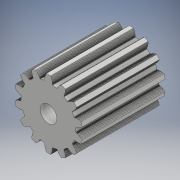
# Autodesk Inventor part: engranaje_pequeño_1
Saved by Autodesk Inventor 2017 (Build 210142000, 142)
## iProperties
Created: 2016-10-04
Part Number: engranaje_pequeño_1
Material: Generic
Document SubType Name: Modeling
Designer: ANDRES
Density: 1 g/cm^3
Appearance: Default
Author: ANDRES
Autodesk Inventor part; units mm, degrees
(part 1 of 2)
ref_plane "YZ Plane" through (0, 0, 0) normal (1, 0, 0) x (0, 1, 0)
ref_plane "XZ Plane" through (0, 0, 0) normal (0, 1, 0) x (-1, 0, 0)
ref_plane "XY Plane" through (0, 0, 0) normal (0, 0, 1) x (1, 0, 0)
sketch "Sketch1" plane through (0, 0, 0) normal (0, 1, 0) x (-1, 0, 0)
  line L0 (0.0808, 0.4341) -> (0.0797, 0.4378)
  line L1 (0.0797, 0.4378) -> (0.0785, 0.4393)
  line L2 (0.0785, 0.4393) -> (0.0772, 0.4404)
  line L3 (0.0772, 0.4404) -> (0.076, 0.4413)
  line L4 (0.076, 0.4413) -> (0.0747, 0.442)
  line L5 (0.0747, 0.442) -> (0.0734, 0.4426)
  line L6 (0.0734, 0.4426) -> (0.0708, 0.4437)
  line L7 (0.0708, 0.4437) -> (0.0682, 0.4445)
  line L8 (0.0682, 0.4445) -> (0.0656, 0.4451)
  line L9 (0.0656, 0.4451) -> (0.0604, 0.4462)
  line L10 (0.0604, 0.4462) -> (0.0552, 0.4478)
  line L11 (0.0552, 0.4478) -> (0.05, 0.4497)
  line L12 (0.05, 0.4497) -> (0.0449, 0.452)
  line L13 (0.0449, 0.452) -> (0.0398, 0.4545)
  line L14 (0.0398, 0.4545) -> (0.0348, 0.4573)
  line L15 (0.0348, 0.4573) -> (0.0298, 0.4603)
  line L16 (0.0298, 0.4603) -> (0.0248, 0.4636)
  line L17 (0.0248, 0.4636) -> (0.0199, 0.467)
  line L18 (0.0199, 0.467) -> (0.015, 0.4707)
  line L19 (0.015, 0.4707) -> (0.0102, 0.4745)
  line L20 (0.0102, 0.4745) -> (0.0055, 0.4786)
  line L21 (0.0055, 0.4786) -> (0.0167, 0.5276)
  line L22 (0.0167, 0.5276) -> (0.0227, 0.5292)
  line L23 (0.0227, 0.5292) -> (0.0287, 0.5306)
  line L24 (0.0287, 0.5306) -> (0.0347, 0.5318)
  line L25 (0.0347, 0.5318) -> (0.0406, 0.5328)
  line L26 (0.0406, 0.5328) -> (0.0465, 0.5335)
  line L27 (0.0465, 0.5335) -> (0.0523, 0.5341)
  line L28 (0.0523, 0.5341) -> (0.058, 0.5344)
  line L29 (0.058, 0.5344) -> (0.0637, 0.5345)
  line L30 (0.0637, 0.5345) -> (0.0693, 0.5343)
  line L31 (0.0693, 0.5343) -> (0.0748, 0.5338)
  line L32 (0.0748, 0.5338) -> (0.0802, 0.5329)
  line L33 (0.0802, 0.5329) -> (0.0854, 0.5316)
  line L34 (0.0854, 0.5316) -> (0.088, 0.5311)
  line L35 (0.088, 0.5311) -> (0.0907, 0.5307)
  line L36 (0.0907, 0.5307) -> (0.0935, 0.5305)
  line L37 (0.0935, 0.5305) -> (0.0949, 0.5305)
  line L38 (0.0949, 0.5305) -> (0.0964, 0.5307)
  line L39 (0.0964, 0.5307) -> (0.0979, 0.5309)
  line L40 (0.0979, 0.5309) -> (0.0995, 0.5313)
  line L41 (0.0995, 0.5313) -> (0.1012, 0.5322)
  line L42 (0.1012, 0.5322) -> (0.1038, 0.535)
  line L43 (0.1038, 0.535) -> (0.1233, 0.5755)
  line L44 (0.1233, 0.5755) -> (0.1239, 0.5792)
  line L45 (0.1239, 0.5792) -> (0.1235, 0.5811)
  line L46 (0.1235, 0.5811) -> (0.1228, 0.5826)
  line L47 (0.1228, 0.5826) -> (0.1221, 0.584)
  line L48 (0.1221, 0.584) -> (0.1212, 0.5852)
  line L49 (0.1212, 0.5852) -> (0.1204, 0.5863)
  line L50 (0.1204, 0.5863) -> (0.1185, 0.5884)
  line L51 (0.1185, 0.5884) -> (0.1165, 0.5903)
  line L52 (0.1165, 0.5903) -> (0.1144, 0.592)
  line L53 (0.1144, 0.592) -> (0.1102, 0.5952)
  line L54 (0.1102, 0.5952) -> (0.1061, 0.5989)
  line L55 (0.1061, 0.5989) -> (0.1023, 0.6029)
  line L56 (0.1023, 0.6029) -> (0.0987, 0.6071)
  line L57 (0.0987, 0.6071) -> (0.0952, 0.6116)
  line L58 (0.0952, 0.6116) -> (0.0919, 0.6163)
  line L59 (0.0919, 0.6163) -> (0.0887, 0.6212)
  line L60 (0.0887, 0.6212) -> (0.0856, 0.6263)
  line L61 (0.0856, 0.6263) -> (0.0827, 0.6315)
  line L62 (0.0827, 0.6315) -> (0.0799, 0.6369)
  line L63 (0.0799, 0.6369) -> (0.0773, 0.6425)
  line L64 (0.0773, 0.6425) -> (0.0747, 0.6482)
  line L65 (0.0747, 0.6482) -> (0.1061, 0.6875)
  line L66 (0.1061, 0.6875) -> (0.1122, 0.6863)
  line L67 (0.1122, 0.6863) -> (0.1182, 0.685)
  line L68 (0.1182, 0.685) -> (0.1241, 0.6835)
  line L69 (0.1241, 0.6835) -> (0.1299, 0.6818)
  line L70 (0.1299, 0.6818) -> (0.1355, 0.6799)
  line L71 (0.1355, 0.6799) -> (0.141, 0.6779)
  line L72 (0.141, 0.6779) -> (0.1463, 0.6757)
  line L73 (0.1463, 0.6757) -> (0.1515, 0.6733)
  line L74 (0.1515, 0.6733) -> (0.1564, 0.6707)
  line L75 (0.1564, 0.6707) -> (0.1612, 0.6679)
  line L76 (0.1612, 0.6679) -> (0.1656, 0.6648)
  line L77 (0.1656, 0.6648) -> (0.1697, 0.6613)
  line L78 (0.1697, 0.6613) -> (0.1719, 0.6597)
  line L79 (0.1719, 0.6597) -> (0.1741, 0.6582)
  line L80 (0.1741, 0.6582) -> (0.1766, 0.6568)
  line L81 (0.1766, 0.6568) -> (0.1779, 0.6562)
  line L82 (0.1779, 0.6562) -> (0.1792, 0.6557)
  line L83 (0.1792, 0.6557) -> (0.1807, 0.6552)
  line L84 (0.1807, 0.6552) -> (0.1823, 0.6549)
  line L85 (0.1823, 0.6549) -> (0.1843, 0.6549)
  line L86 (0.1843, 0.6549) -> (0.1878, 0.6564)
  line L87 (0.1878, 0.6564) -> (0.2229, 0.6844)
  line L88 (0.2229, 0.6844) -> (0.2251, 0.6875)
  line L89 (0.2251, 0.6875) -> (0.2255, 0.6894)
  line L90 (0.2255, 0.6894) -> (0.2256, 0.691)
  line L91 (0.2256, 0.691) -> (0.2255, 0.6926)
  line L92 (0.2255, 0.6926) -> (0.2253, 0.694)
  line L93 (0.2253, 0.694) -> (0.225, 0.6954)
  line L94 (0.225, 0.6954) -> (0.2242, 0.6981)
  line L95 (0.2242, 0.6981) -> (0.2232, 0.7006)
  line L96 (0.2232, 0.7006) -> (0.2221, 0.7031)
  line L97 (0.2221, 0.7031) -> (0.2197, 0.7079)
  line L98 (0.2197, 0.7079) -> (0.2176, 0.7129)
  line L99 (0.2176, 0.7129) -> (0.2159, 0.7182)
  line L100 (0.2159, 0.7182) -> (0.2145, 0.7236)
  line L101 (0.2145, 0.7236) -> (0.2133, 0.7291)
  line L102 (0.2133, 0.7291) -> (0.2123, 0.7348)
  line L103 (0.2123, 0.7348) -> (0.2116, 0.7406)
  line L104 (0.2116, 0.7406) -> (0.211, 0.7465)
  line L105 (0.211, 0.7465) -> (0.2107, 0.7525)
  line L106 (0.2107, 0.7525) -> (0.2105, 0.7586)
  line L107 (0.2105, 0.7586) -> (0.2105, 0.7647)
  line L108 (0.2105, 0.7647) -> (0.2107, 0.771)
  line L109 (0.2107, 0.771) -> (0.256, 0.7928)
  line L110 (0.256, 0.7928) -> (0.261, 0.7891)
  line L111 (0.261, 0.7891) -> (0.2659, 0.7852)
  line L112 (0.2659, 0.7852) -> (0.2705, 0.7813)
  line L113 (0.2705, 0.7813) -> (0.275, 0.7773)
  line L114 (0.275, 0.7773) -> (0.2793, 0.7732)
  line L115 (0.2793, 0.7732) -> (0.2833, 0.769)
  line L116 (0.2833, 0.769) -> (0.2872, 0.7647)
  line L117 (0.2872, 0.7647) -> (0.2908, 0.7603)
  line L118 (0.2908, 0.7603) -> (0.2941, 0.7558)
  line L119 (0.2941, 0.7558) -> (0.2971, 0.7512)
  line L120 (0.2971, 0.7512) -> (0.2998, 0.7465)
  line L121 (0.2998, 0.7465) -> (0.302, 0.7416)
  line L122 (0.302, 0.7416) -> (0.3032, 0.7392)
  line L123 (0.3032, 0.7392) -> (0.3046, 0.7368)
  line L124 (0.3046, 0.7368) -> (0.3062, 0.7345)
  line L125 (0.3062, 0.7345) -> (0.3071, 0.7334)
  line L126 (0.3071, 0.7334) -> (0.3081, 0.7323)
  line L127 (0.3081, 0.7323) -> (0.3093, 0.7313)
  line L128 (0.3093, 0.7313) -> (0.3106, 0.7304)
  line L129 (0.3106, 0.7304) -> (0.3123, 0.7295)
  line L130 (0.3123, 0.7295) -> (0.3161, 0.7293)
  line L131 (0.3161, 0.7293) -> (0.3599, 0.7393)
  line L132 (0.3599, 0.7393) -> (0.3633, 0.7411)
  line L133 (0.3633, 0.7411) -> (0.3644, 0.7426)
  line L134 (0.3644, 0.7426) -> (0.3652, 0.7441)
  line L135 (0.3652, 0.7441) -> (0.3658, 0.7455)
  line L136 (0.3658, 0.7455) -> (0.3663, 0.7469)
  line L137 (0.3663, 0.7469) -> (0.3666, 0.7483)
  line L138 (0.3666, 0.7483) -> (0.367, 0.7511)
  line L139 (0.367, 0.7511) -> (0.3673, 0.7538)
  line L140 (0.3673, 0.7538) -> (0.3673, 0.7565)
  line L141 (0.3673, 0.7565) -> (0.3672, 0.7618)
  line L142 (0.3672, 0.7618) -> (0.3676, 0.7673)
  line L143 (0.3676, 0.7673) -> (0.3683, 0.7727)
  line L144 (0.3683, 0.7727) -> (0.3694, 0.7782)
  line L145 (0.3694, 0.7782) -> (0.3707, 0.7837)
  line L146 (0.3707, 0.7837) -> (0.3723, 0.7893)
  line L147 (0.3723, 0.7893) -> (0.3741, 0.7948)
  line L148 (0.3741, 0.7948) -> (0.3762, 0.8004)
  line L149 (0.3762, 0.8004) -> (0.3784, 0.8059)
  line L150 (0.3784, 0.8059) -> (0.3809, 0.8115)
  line L151 (0.3809, 0.8115) -> (0.3836, 0.817)
  line L152 (0.3836, 0.817) -> (0.3865, 0.8226)
  line L153 (0.3865, 0.8226) -> (0.4368, 0.8226)
  line L154 (0.4368, 0.8226) -> (0.4397, 0.817)
  line L155 (0.4397, 0.817) -> (0.4424, 0.8115)
  line L156 (0.4424, 0.8115) -> (0.4449, 0.8059)
  line L157 (0.4449, 0.8059) -> (0.4472, 0.8004)
  line L158 (0.4472, 0.8004) -> (0.4492, 0.7948)
  line L159 (0.4492, 0.7948) -> (0.4511, 0.7893)
  line L160 (0.4511, 0.7893) -> (0.4526, 0.7837)
  line L161 (0.4526, 0.7837) -> (0.454, 0.7782)
  line L162 (0.454, 0.7782) -> (0.455, 0.7727)
  line L163 (0.455, 0.7727) -> (0.4558, 0.7673)
  line L164 (0.4558, 0.7673) -> (0.4561, 0.7618)
  line L165 (0.4561, 0.7618) -> (0.456, 0.7565)
  line L166 (0.456, 0.7565) -> (0.4561, 0.7538)
  line L167 (0.4561, 0.7538) -> (0.4563, 0.7511)
  line L168 (0.4563, 0.7511) -> (0.4567, 0.7483)
  line L169 (0.4567, 0.7483) -> (0.4571, 0.7469)
  line L170 (0.4571, 0.7469) -> (0.4575, 0.7455)
  line L171 (0.4575, 0.7455) -> (0.4581, 0.7441)
  line L172 (0.4581, 0.7441) -> (0.4589, 0.7426)
  line L173 (0.4589, 0.7426) -> (0.4601, 0.7411)
  line L174 (0.4601, 0.7411) -> (0.4634, 0.7393)
  line L175 (0.4634, 0.7393) -> (0.5072, 0.7293)
  line L176 (0.5072, 0.7293) -> (0.511, 0.7295)
  line L177 (0.511, 0.7295) -> (0.5127, 0.7304)
  line L178 (0.5127, 0.7304) -> (0.5141, 0.7313)
  line L179 (0.5141, 0.7313) -> (0.5152, 0.7323)
  line L180 (0.5152, 0.7323) -> (0.5162, 0.7334)
  line L181 (0.5162, 0.7334) -> (0.5171, 0.7345)
  line L182 (0.5171, 0.7345) -> (0.5187, 0.7368)
  line L183 (0.5187, 0.7368) -> (0.5201, 0.7392)
  line L184 (0.5201, 0.7392) -> (0.5213, 0.7416)
  line L185 (0.5213, 0.7416) -> (0.5235, 0.7465)
  line L186 (0.5235, 0.7465) -> (0.5262, 0.7512)
  line L187 (0.5262, 0.7512) -> (0.5292, 0.7558)
  line L188 (0.5292, 0.7558) -> (0.5326, 0.7603)
  line L189 (0.5326, 0.7603) -> (0.5362, 0.7647)
  line L190 (0.5362, 0.7647) -> (0.54, 0.769)
  line L191 (0.54, 0.769) -> (0.5441, 0.7732)
  line L192 (0.5441, 0.7732) -> (0.5483, 0.7773)
  line L193 (0.5483, 0.7773) -> (0.5528, 0.7813)
  line L194 (0.5528, 0.7813) -> (0.5575, 0.7852)
  line L195 (0.5575, 0.7852) -> (0.5623, 0.7891)
  line L196 (0.5623, 0.7891) -> (0.5673, 0.7928)
  line L197 (0.5673, 0.7928) -> (0.6126, 0.771)
  line L198 (0.6126, 0.771) -> (0.6128, 0.7647)
  line L199 (0.6128, 0.7647) -> (0.6128, 0.7586)
  line L200 (0.6128, 0.7586) -> (0.6127, 0.7525)
  line L201 (0.6127, 0.7525) -> (0.6123, 0.7465)
  line L202 (0.6123, 0.7465) -> (0.6118, 0.7406)
  line L203 (0.6118, 0.7406) -> (0.611, 0.7348)
  line L204 (0.611, 0.7348) -> (0.61, 0.7291)
  line L205 (0.61, 0.7291) -> (0.6088, 0.7236)
  line L206 (0.6088, 0.7236) -> (0.6074, 0.7182)
  line L207 (0.6074, 0.7182) -> (0.6057, 0.7129)
  line L208 (0.6057, 0.7129) -> (0.6037, 0.7079)
  line L209 (0.6037, 0.7079) -> (0.6012, 0.7031)
  line L210 (0.6012, 0.7031) -> (0.6001, 0.7006)
  line L211 (0.6001, 0.7006) -> (0.5991, 0.6981)
  line L212 (0.5991, 0.6981) -> (0.5983, 0.6954)
  line L213 (0.5983, 0.6954) -> (0.598, 0.694)
  line L214 (0.598, 0.694) -> (0.5978, 0.6926)
  line L215 (0.5978, 0.6926) -> (0.5977, 0.691)
  line L216 (0.5977, 0.691) -> (0.5978, 0.6894)
  line L217 (0.5978, 0.6894) -> (0.5982, 0.6875)
  line L218 (0.5982, 0.6875) -> (0.6004, 0.6844)
  line L219 (0.6004, 0.6844) -> (0.6355, 0.6564)
  line L220 (0.6355, 0.6564) -> (0.6391, 0.6549)
  line L221 (0.6391, 0.6549) -> (0.641, 0.6549)
  line L222 (0.641, 0.6549) -> (0.6426, 0.6552)
  line L223 (0.6426, 0.6552) -> (0.6441, 0.6557)
  line L224 (0.6441, 0.6557) -> (0.6455, 0.6562)
  line L225 (0.6455, 0.6562) -> (0.6468, 0.6568)
  line L226 (0.6468, 0.6568) -> (0.6492, 0.6582)
  line L227 (0.6492, 0.6582) -> (0.6515, 0.6597)
  line L228 (0.6515, 0.6597) -> (0.6536, 0.6613)
  line L229 (0.6536, 0.6613) -> (0.6577, 0.6648)
  line L230 (0.6577, 0.6648) -> (0.6622, 0.6679)
  line L231 (0.6622, 0.6679) -> (0.6669, 0.6707)
  line L232 (0.6669, 0.6707) -> (0.6719, 0.6733)
  line L233 (0.6719, 0.6733) -> (0.677, 0.6757)
  line L234 (0.677, 0.6757) -> (0.6823, 0.6779)
  line L235 (0.6823, 0.6779) -> (0.6878, 0.6799)
  line L236 (0.6878, 0.6799) -> (0.6934, 0.6818)
  line L237 (0.6934, 0.6818) -> (0.6992, 0.6835)
  line L238 (0.6992, 0.6835) -> (0.7051, 0.685)
  line L239 (0.7051, 0.685) -> (0.7111, 0.6863)
  line L240 (0.7111, 0.6863) -> (0.7172, 0.6875)
  line L241 (0.7172, 0.6875) -> (0.7486, 0.6482)
  line L242 (0.7486, 0.6482) -> (0.7461, 0.6425)
  line L243 (0.7461, 0.6425) -> (0.7434, 0.6369)
  line L244 (0.7434, 0.6369) -> (0.7406, 0.6315)
  line L245 (0.7406, 0.6315) -> (0.7377, 0.6263)
  line L246 (0.7377, 0.6263) -> (0.7347, 0.6212)
  line L247 (0.7347, 0.6212) -> (0.7315, 0.6163)
  line L248 (0.7315, 0.6163) -> (0.7281, 0.6116)
  line L249 (0.7281, 0.6116) -> (0.7246, 0.6071)
  line L250 (0.7246, 0.6071) -> (0.721, 0.6029)
  line L251 (0.721, 0.6029) -> (0.7172, 0.5989)
  line L252 (0.7172, 0.5989) -> (0.7132, 0.5952)
  line L253 (0.7132, 0.5952) -> (0.7089, 0.592)
  line L254 (0.7089, 0.592) -> (0.7068, 0.5903)
  line L255 (0.7068, 0.5903) -> (0.7048, 0.5884)
  line L256 (0.7048, 0.5884) -> (0.703, 0.5863)
  line L257 (0.703, 0.5863) -> (0.7021, 0.5852)
  line L258 (0.7021, 0.5852) -> (0.7013, 0.584)
  line L259 (0.7013, 0.584) -> (0.7005, 0.5826)
  line L260 (0.7005, 0.5826) -> (0.6999, 0.5811)
  line L261 (0.6999, 0.5811) -> (0.6994, 0.5792)
  line L262 (0.6994, 0.5792) -> (0.7, 0.5755)
  line L263 (0.7, 0.5755) -> (0.7195, 0.535)
  line L264 (0.7195, 0.535) -> (0.7221, 0.5322)
  line L265 (0.7221, 0.5322) -> (0.7238, 0.5313)
  line L266 (0.7238, 0.5313) -> (0.7254, 0.5309)
  line L267 (0.7254, 0.5309) -> (0.7269, 0.5307)
  line L268 (0.7269, 0.5307) -> (0.7284, 0.5305)
  line L269 (0.7284, 0.5305) -> (0.7299, 0.5305)
  line L270 (0.7299, 0.5305) -> (0.7326, 0.5307)
  line L271 (0.7326, 0.5307) -> (0.7353, 0.5311)
  line L272 (0.7353, 0.5311) -> (0.738, 0.5316)
  line L273 (0.738, 0.5316) -> (0.7432, 0.5329)
  line L274 (0.7432, 0.5329) -> (0.7485, 0.5338)
  line L275 (0.7485, 0.5338) -> (0.754, 0.5343)
  line L276 (0.754, 0.5343) -> (0.7596, 0.5345)
  line L277 (0.7596, 0.5345) -> (0.7653, 0.5344)
  line L278 (0.7653, 0.5344) -> (0.771, 0.5341)
  line L279 (0.771, 0.5341) -> (0.7769, 0.5335)
  line L280 (0.7769, 0.5335) -> (0.7827, 0.5328)
  line L281 (0.7827, 0.5328) -> (0.7887, 0.5318)
  line L282 (0.7887, 0.5318) -> (0.7946, 0.5306)
  line L283 (0.7946, 0.5306) -> (0.8006, 0.5292)
  line L284 (0.8006, 0.5292) -> (0.8067, 0.5276)
  line L285 (0.8067, 0.5276) -> (0.8178, 0.4786)
  line L286 (0.8178, 0.4786) -> (0.8131, 0.4745)
  line L287 (0.8131, 0.4745) -> (0.8083, 0.4707)
  line L288 (0.8083, 0.4707) -> (0.8034, 0.467)
  line L289 (0.8034, 0.467) -> (0.7985, 0.4636)
  line L290 (0.7985, 0.4636) -> (0.7936, 0.4603)
  line L291 (0.7936, 0.4603) -> (0.7886, 0.4573)
  line L292 (0.7886, 0.4573) -> (0.7835, 0.4545)
  line L293 (0.7835, 0.4545) -> (0.7784, 0.452)
  line L294 (0.7784, 0.452) -> (0.7733, 0.4497)
  line L295 (0.7733, 0.4497) -> (0.7682, 0.4478)
  line L296 (0.7682, 0.4478) -> (0.763, 0.4462)
  line L297 (0.763, 0.4462) -> (0.7577, 0.4451)
  line L298 (0.7577, 0.4451) -> (0.7551, 0.4445)
  line L299 (0.7551, 0.4445) -> (0.7525, 0.4437)
  line L300 (0.7525, 0.4437) -> (0.7499, 0.4426)
  line L301 (0.7499, 0.4426) -> (0.7486, 0.442)
  line L302 (0.7486, 0.442) -> (0.7473, 0.4413)
  line L303 (0.7473, 0.4413) -> (0.7461, 0.4404)
  line L304 (0.7461, 0.4404) -> (0.7449, 0.4393)
  line L305 (0.7449, 0.4393) -> (0.7436, 0.4378)
  line L306 (0.7436, 0.4378) -> (0.7426, 0.4341)
  line L307 (0.7426, 0.4341) -> (0.7426, 0.3892)
  line L308 (0.7426, 0.3892) -> (0.7436, 0.3855)
  line L309 (0.7436, 0.3855) -> (0.7449, 0.3841)
  line L310 (0.7449, 0.3841) -> (0.7461, 0.383)
  line L311 (0.7461, 0.383) -> (0.7473, 0.3821)
  line L312 (0.7473, 0.3821) -> (0.7486, 0.3813)
  line L313 (0.7486, 0.3813) -> (0.7499, 0.3807)
  line L314 (0.7499, 0.3807) -> (0.7525, 0.3796)
  line L315 (0.7525, 0.3796) -> (0.7551, 0.3788)
  line L316 (0.7551, 0.3788) -> (0.7577, 0.3782)
  line L317 (0.7577, 0.3782) -> (0.763, 0.3771)
  line L318 (0.763, 0.3771) -> (0.7682, 0.3755)
  line L319 (0.7682, 0.3755) -> (0.7733, 0.3736)
  line L320 (0.7733, 0.3736) -> (0.7784, 0.3714)
  line L321 (0.7784, 0.3714) -> (0.7835, 0.3688)
  line L322 (0.7835, 0.3688) -> (0.7886, 0.366)
  line L323 (0.7886, 0.366) -> (0.7936, 0.363)
  line L324 (0.7936, 0.363) -> (0.7985, 0.3598)
  line L325 (0.7985, 0.3598) -> (0.8034, 0.3563)
  line L326 (0.8034, 0.3563) -> (0.8083, 0.3527)
  line L327 (0.8083, 0.3527) -> (0.8131, 0.3488)
  line L328 (0.8131, 0.3488) -> (0.8178, 0.3447)
  line L329 (0.8178, 0.3447) -> (0.8067, 0.2957)
  line L330 (0.8067, 0.2957) -> (0.8006, 0.2941)
  line L331 (0.8006, 0.2941) -> (0.7946, 0.2927)
  line L332 (0.7946, 0.2927) -> (0.7887, 0.2915)
  line L333 (0.7887, 0.2915) -> (0.7827, 0.2906)
  line L334 (0.7827, 0.2906) -> (0.7769, 0.2898)
  line L335 (0.7769, 0.2898) -> (0.771, 0.2892)
  line L336 (0.771, 0.2892) -> (0.7653, 0.2889)
  line L337 (0.7653, 0.2889) -> (0.7596, 0.2888)
  line L338 (0.7596, 0.2888) -> (0.754, 0.289)
  line L339 (0.754, 0.289) -> (0.7485, 0.2895)
  line L340 (0.7485, 0.2895) -> (0.7432, 0.2904)
  line L341 (0.7432, 0.2904) -> (0.738, 0.2917)
  line L342 (0.738, 0.2917) -> (0.7353, 0.2923)
  line L343 (0.7353, 0.2923) -> (0.7326, 0.2927)
  line L344 (0.7326, 0.2927) -> (0.7299, 0.2928)
  line L345 (0.7299, 0.2928) -> (0.7284, 0.2928)
  line L346 (0.7284, 0.2928) -> (0.7269, 0.2927)
  line L347 (0.7269, 0.2927) -> (0.7254, 0.2924)
  line L348 (0.7254, 0.2924) -> (0.7238, 0.292)
  line L349 (0.7238, 0.292) -> (0.7221, 0.2912)
  line L350 (0.7221, 0.2912) -> (0.7195, 0.2883)
  line L351 (0.7195, 0.2883) -> (0.7, 0.2479)
  line L352 (0.7, 0.2479) -> (0.6994, 0.2441)
  line L353 (0.6994, 0.2441) -> (0.6999, 0.2422)
  line L354 (0.6999, 0.2422) -> (0.7005, 0.2407)
  line L355 (0.7005, 0.2407) -> (0.7013, 0.2394)
  line L356 (0.7013, 0.2394) -> (0.7021, 0.2381)
  line L357 (0.7021, 0.2381) -> (0.703, 0.237)
  line L358 (0.703, 0.237) -> (0.7048, 0.2349)
  line L359 (0.7048, 0.2349) -> (0.7068, 0.2331)
  line L360 (0.7068, 0.2331) -> (0.7089, 0.2314)
  line L361 (0.7089, 0.2314) -> (0.7132, 0.2281)
  line L362 (0.7132, 0.2281) -> (0.7172, 0.2244)
  line L363 (0.7172, 0.2244) -> (0.721, 0.2205)
  line L364 (0.721, 0.2205) -> (0.7246, 0.2162)
  line L365 (0.7246, 0.2162) -> (0.7281, 0.2117)
  line L366 (0.7281, 0.2117) -> (0.7315, 0.207)
  line L367 (0.7315, 0.207) -> (0.7347, 0.2021)
  line L368 (0.7347, 0.2021) -> (0.7377, 0.1971)
  line L369 (0.7377, 0.1971) -> (0.7406, 0.1918)
  line L370 (0.7406, 0.1918) -> (0.7434, 0.1864)
  line L371 (0.7434, 0.1864) -> (0.7461, 0.1809)
  line L372 (0.7461, 0.1809) -> (0.7486, 0.1751)
  line L373 (0.7486, 0.1751) -> (0.7172, 0.1358)
  line L374 (0.7172, 0.1358) -> (0.7111, 0.137)
  line L375 (0.7111, 0.137) -> (0.7051, 0.1384)
  line L376 (0.7051, 0.1384) -> (0.6992, 0.1399)
  line L377 (0.6992, 0.1399) -> (0.6934, 0.1416)
  line L378 (0.6934, 0.1416) -> (0.6878, 0.1434)
  line L379 (0.6878, 0.1434) -> (0.6823, 0.1454)
  line L380 (0.6823, 0.1454) -> (0.677, 0.1476)
  line L381 (0.677, 0.1476) -> (0.6719, 0.15)
  line L382 (0.6719, 0.15) -> (0.6669, 0.1526)
  line L383 (0.6669, 0.1526) -> (0.6622, 0.1555)
  line L384 (0.6622, 0.1555) -> (0.6577, 0.1586)
  line L385 (0.6577, 0.1586) -> (0.6536, 0.162)
  line L386 (0.6536, 0.162) -> (0.6515, 0.1637)
  line L387 (0.6515, 0.1637) -> (0.6492, 0.1652)
  line L388 (0.6492, 0.1652) -> (0.6468, 0.1665)
  line L389 (0.6468, 0.1665) -> (0.6455, 0.1671)
  line L390 (0.6455, 0.1671) -> (0.6441, 0.1677)
  line L391 (0.6441, 0.1677) -> (0.6426, 0.1681)
  line L392 (0.6426, 0.1681) -> (0.641, 0.1684)
  line L393 (0.641, 0.1684) -> (0.6391, 0.1684)
  line L394 (0.6391, 0.1684) -> (0.6355, 0.167)
  line L395 (0.6355, 0.167) -> (0.6004, 0.1389)
  line L396 (0.6004, 0.1389) -> (0.5982, 0.1358)
  line L397 (0.5982, 0.1358) -> (0.5978, 0.134)
  line L398 (0.5978, 0.134) -> (0.5977, 0.1323)
  line L399 (0.5977, 0.1323) -> (0.5978, 0.1308)
  line L400 (0.5978, 0.1308) -> (0.598, 0.1293)
  line L401 (0.598, 0.1293) -> (0.5983, 0.1279)
  line L402 (0.5983, 0.1279) -> (0.5991, 0.1252)
  line L403 (0.5991, 0.1252) -> (0.6001, 0.1227)
  line L404 (0.6001, 0.1227) -> (0.6012, 0.1203)
  line L405 (0.6012, 0.1203) -> (0.6037, 0.1155)
  line L406 (0.6037, 0.1155) -> (0.6057, 0.1104)
  line L407 (0.6057, 0.1104) -> (0.6074, 0.1052)
  line L408 (0.6074, 0.1052) -> (0.6088, 0.0998)
  line L409 (0.6088, 0.0998) -> (0.61, 0.0942)
  line L410 (0.61, 0.0942) -> (0.611, 0.0885)
  line L411 (0.611, 0.0885) -> (0.6118, 0.0828)
  line L412 (0.6118, 0.0828) -> (0.6123, 0.0769)
  line L413 (0.6123, 0.0769) -> (0.6127, 0.0709)
  line L414 (0.6127, 0.0709) -> (0.6128, 0.0648)
  line L415 (0.6128, 0.0648) -> (0.6128, 0.0586)
  line L416 (0.6128, 0.0586) -> (0.6126, 0.0524)
  line L417 (0.6126, 0.0524) -> (0.5673, 0.0306)
  line L418 (0.5673, 0.0306) -> (0.5623, 0.0343)
  line L419 (0.5623, 0.0343) -> (0.5575, 0.0381)
  line L420 (0.5575, 0.0381) -> (0.5528, 0.042)
  line L421 (0.5528, 0.042) -> (0.5483, 0.046)
  line L422 (0.5483, 0.046) -> (0.5441, 0.0502)
  line L423 (0.5441, 0.0502) -> (0.54, 0.0544)
  line L424 (0.54, 0.0544) -> (0.5362, 0.0587)
  line L425 (0.5362, 0.0587) -> (0.5326, 0.063)
  line L426 (0.5326, 0.063) -> (0.5292, 0.0675)
  line L427 (0.5292, 0.0675) -> (0.5262, 0.0721)
  line L428 (0.5262, 0.0721) -> (0.5235, 0.0769)
  line L429 (0.5235, 0.0769) -> (0.5213, 0.0818)
  line L430 (0.5213, 0.0818) -> (0.5201, 0.0842)
  line L431 (0.5201, 0.0842) -> (0.5187, 0.0865)
  line L432 (0.5187, 0.0865) -> (0.5171, 0.0888)
  line L433 (0.5171, 0.0888) -> (0.5162, 0.0899)
  line L434 (0.5162, 0.0899) -> (0.5152, 0.091)
  line L435 (0.5152, 0.091) -> (0.5141, 0.092)
  line L436 (0.5141, 0.092) -> (0.5127, 0.093)
  line L437 (0.5127, 0.093) -> (0.511, 0.0938)
  line L438 (0.511, 0.0938) -> (0.5072, 0.0941)
  line L439 (0.5072, 0.0941) -> (0.4634, 0.0841)
  line L440 (0.4634, 0.0841) -> (0.4601, 0.0822)
  line L441 (0.4601, 0.0822) -> (0.4589, 0.0807)
  line L442 (0.4589, 0.0807) -> (0.4581, 0.0792)
  line L443 (0.4581, 0.0792) -> (0.4575, 0.0778)
  line L444 (0.4575, 0.0778) -> (0.4571, 0.0764)
  line L445 (0.4571, 0.0764) -> (0.4567, 0.075)
  line L446 (0.4567, 0.075) -> (0.4563, 0.0723)
  line L447 (0.4563, 0.0723) -> (0.4561, 0.0695)
  line L448 (0.4561, 0.0695) -> (0.456, 0.0669)
  line L449 (0.456, 0.0669) -> (0.4561, 0.0615)
  line L450 (0.4561, 0.0615) -> (0.4558, 0.0561)
  line L451 (0.4558, 0.0561) -> (0.455, 0.0506)
  line L452 (0.455, 0.0506) -> (0.454, 0.0451)
  line L453 (0.454, 0.0451) -> (0.4526, 0.0396)
  line L454 (0.4526, 0.0396) -> (0.4511, 0.034)
  line L455 (0.4511, 0.034) -> (0.4492, 0.0285)
  line L456 (0.4492, 0.0285) -> (0.4472, 0.023)
  line L457 (0.4472, 0.023) -> (0.4449, 0.0174)
  line L458 (0.4449, 0.0174) -> (0.4424, 0.0119)
  line L459 (0.4424, 0.0119) -> (0.4397, 0.0063)
  line L460 (0.4397, 0.0063) -> (0.4368, 0.0008)
  line L461 (0.4368, 0.0008) -> (0.3865, 0.0008)
  line L462 (0.3865, 0.0008) -> (0.3836, 0.0063)
  line L463 (0.3836, 0.0063) -> (0.3809, 0.0119)
  line L464 (0.3809, 0.0119) -> (0.3784, 0.0174)
  line L465 (0.3784, 0.0174) -> (0.3762, 0.023)
  line L466 (0.3762, 0.023) -> (0.3741, 0.0285)
  line L467 (0.3741, 0.0285) -> (0.3723, 0.034)
  line L468 (0.3723, 0.034) -> (0.3707, 0.0396)
  line L469 (0.3707, 0.0396) -> (0.3694, 0.0451)
  line L470 (0.3694, 0.0451) -> (0.3683, 0.0506)
  line L471 (0.3683, 0.0506) -> (0.3676, 0.0561)
  line L472 (0.3676, 0.0561) -> (0.3672, 0.0615)
  line L473 (0.3672, 0.0615) -> (0.3673, 0.0669)
  line L474 (0.3673, 0.0669) -> (0.3673, 0.0695)
  line L475 (0.3673, 0.0695) -> (0.367, 0.0723)
  line L476 (0.367, 0.0723) -> (0.3666, 0.075)
  line L477 (0.3666, 0.075) -> (0.3663, 0.0764)
  line L478 (0.3663, 0.0764) -> (0.3658, 0.0778)
  line L479 (0.3658, 0.0778) -> (0.3652, 0.0792)
  line L480 (0.3652, 0.0792) -> (0.3644, 0.0807)
  line L481 (0.3644, 0.0807) -> (0.3633, 0.0822)
  line L482 (0.3633, 0.0822) -> (0.3599, 0.0841)
  line L483 (0.3599, 0.0841) -> (0.3161, 0.0941)
  line L484 (0.3161, 0.0941) -> (0.3123, 0.0938)
  line L485 (0.3123, 0.0938) -> (0.3106, 0.093)
  line L486 (0.3106, 0.093) -> (0.3093, 0.092)
  line L487 (0.3093, 0.092) -> (0.3081, 0.091)
  line L488 (0.3081, 0.091) -> (0.3071, 0.0899)
  line L489 (0.3071, 0.0899) -> (0.3062, 0.0888)
  line L490 (0.3062, 0.0888) -> (0.3046, 0.0865)
  line L491 (0.3046, 0.0865) -> (0.3032, 0.0842)
  line L492 (0.3032, 0.0842) -> (0.302, 0.0818)
  line L493 (0.302, 0.0818) -> (0.2998, 0.0769)
  line L494 (0.2998, 0.0769) -> (0.2971, 0.0721)
  line L495 (0.2971, 0.0721) -> (0.2941, 0.0675)
  line L496 (0.2941, 0.0675) -> (0.2908, 0.063)
  line L497 (0.2908, 0.063) -> (0.2872, 0.0587)
  line L498 (0.2872, 0.0587) -> (0.2833, 0.0544)
  line L499 (0.2833, 0.0544) -> (0.2793, 0.0502)
  line L500 (0.2793, 0.0502) -> (0.275, 0.046)
  line L501 (0.275, 0.046) -> (0.2705, 0.042)
  line L502 (0.2705, 0.042) -> (0.2659, 0.0381)
  line L503 (0.2659, 0.0381) -> (0.261, 0.0343)
  line L504 (0.261, 0.0343) -> (0.256, 0.0306)
  line L505 (0.256, 0.0306) -> (0.2107, 0.0524)
  line L506 (0.2107, 0.0524) -> (0.2105, 0.0586)
  line L507 (0.2105, 0.0586) -> (0.2105, 0.0648)
  line L508 (0.2105, 0.0648) -> (0.2107, 0.0709)
  line L509 (0.2107, 0.0709) -> (0.211, 0.0769)
  line L510 (0.211, 0.0769) -> (0.2116, 0.0828)
  line L511 (0.2116, 0.0828) -> (0.2123, 0.0885)
  line L512 (0.2123, 0.0885) -> (0.2133, 0.0942)
  line L513 (0.2133, 0.0942) -> (0.2145, 0.0998)
  line L514 (0.2145, 0.0998) -> (0.2159, 0.1052)
  line L515 (0.2159, 0.1052) -> (0.2176, 0.1104)
  line L516 (0.2176, 0.1104) -> (0.2197, 0.1155)
  line L517 (0.2197, 0.1155) -> (0.2221, 0.1203)
  line L518 (0.2221, 0.1203) -> (0.2232, 0.1227)
  line L519 (0.2232, 0.1227) -> (0.2242, 0.1252)
  line L520 (0.2242, 0.1252) -> (0.225, 0.1279)
  line L521 (0.225, 0.1279) -> (0.2253, 0.1293)
  line L522 (0.2253, 0.1293) -> (0.2255, 0.1308)
  line L523 (0.2255, 0.1308) -> (0.2256, 0.1323)
  line L524 (0.2256, 0.1323) -> (0.2255, 0.134)
  line L525 (0.2255, 0.134) -> (0.2251, 0.1358)
  line L526 (0.2251, 0.1358) -> (0.2229, 0.1389)
  line L527 (0.2229, 0.1389) -> (0.1878, 0.167)
  line L528 (0.1878, 0.167) -> (0.1843, 0.1684)
  line L529 (0.1843, 0.1684) -> (0.1823, 0.1684)
  line L530 (0.1823, 0.1684) -> (0.1807, 0.1681)
  line L531 (0.1807, 0.1681) -> (0.1792, 0.1677)
  line L532 (0.1792, 0.1677) -> (0.1779, 0.1671)
  line L533 (0.1779, 0.1671) -> (0.1766, 0.1665)
  line L534 (0.1766, 0.1665) -> (0.1741, 0.1652)
  line L535 (0.1741, 0.1652) -> (0.1719, 0.1637)
  line L536 (0.1719, 0.1637) -> (0.1697, 0.162)
  line L537 (0.1697, 0.162) -> (0.1656, 0.1586)
  line L538 (0.1656, 0.1586) -> (0.1612, 0.1555)
  line L539 (0.1612, 0.1555) -> (0.1564, 0.1526)
  line L540 (0.1564, 0.1526) -> (0.1515, 0.15)
  line L541 (0.1515, 0.15) -> (0.1463, 0.1476)
  line L542 (0.1463, 0.1476) -> (0.141, 0.1454)
  line L543 (0.141, 0.1454) -> (0.1355, 0.1434)
  line L544 (0.1355, 0.1434) -> (0.1299, 0.1416)
  line L545 (0.1299, 0.1416) -> (0.1241, 0.1399)
  line L546 (0.1241, 0.1399) -> (0.1182, 0.1384)
  line L547 (0.1182, 0.1384) -> (0.1122, 0.137)
  line L548 (0.1122, 0.137) -> (0.1061, 0.1358)
  line L549 (0.1061, 0.1358) -> (0.0747, 0.1751)
  line L550 (0.0747, 0.1751) -> (0.0773, 0.1809)
  line L551 (0.0773, 0.1809) -> (0.0799, 0.1864)
  line L552 (0.0799, 0.1864) -> (0.0827, 0.1918)
  line L553 (0.0827, 0.1918) -> (0.0856, 0.1971)
  line L554 (0.0856, 0.1971) -> (0.0887, 0.2021)
  line L555 (0.0887, 0.2021) -> (0.0919, 0.207)
  line L556 (0.0919, 0.207) -> (0.0952, 0.2117)
  line L557 (0.0952, 0.2117) -> (0.0987, 0.2162)
  line L558 (0.0987, 0.2162) -> (0.1023, 0.2205)
  line L559 (0.1023, 0.2205) -> (0.1061, 0.2244)
  line L560 (0.1061, 0.2244) -> (0.1102, 0.2281)
  line L561 (0.1102, 0.2281) -> (0.1144, 0.2314)
  line L562 (0.1144, 0.2314) -> (0.1165, 0.2331)
  line L563 (0.1165, 0.2331) -> (0.1185, 0.2349)
  line L564 (0.1185, 0.2349) -> (0.1204, 0.237)
  line L565 (0.1204, 0.237) -> (0.1212, 0.2381)
  line L566 (0.1212, 0.2381) -> (0.1221, 0.2394)
  line L567 (0.1221, 0.2394) -> (0.1228, 0.2407)
  line L568 (0.1228, 0.2407) -> (0.1235, 0.2422)
  line L569 (0.1235, 0.2422) -> (0.1239, 0.2441)
  line L570 (0.1239, 0.2441) -> (0.1233, 0.2479)
  line L571 (0.1233, 0.2479) -> (0.1038, 0.2883)
  line L572 (0.1038, 0.2883) -> (0.1012, 0.2912)
  line L573 (0.1012, 0.2912) -> (0.0995, 0.292)
  line L574 (0.0995, 0.292) -> (0.0979, 0.2924)
  line L575 (0.0979, 0.2924) -> (0.0964, 0.2927)
  line L576 (0.0964, 0.2927) -> (0.0949, 0.2928)
  line L577 (0.0949, 0.2928) -> (0.0935, 0.2928)
  line L578 (0.0935, 0.2928) -> (0.0907, 0.2927)
  line L579 (0.0907, 0.2927) -> (0.088, 0.2923)
  line L580 (0.088, 0.2923) -> (0.0854, 0.2917)
  line L581 (0.0854, 0.2917) -> (0.0802, 0.2904)
  line L582 (0.0802, 0.2904) -> (0.0748, 0.2895)
  line L583 (0.0748, 0.2895) -> (0.0693, 0.289)
  line L584 (0.0693, 0.289) -> (0.0637, 0.2888)
  line L585 (0.0637, 0.2888) -> (0.058, 0.2889)
  line L586 (0.058, 0.2889) -> (0.0523, 0.2892)
  line L587 (0.0523, 0.2892) -> (0.0465, 0.2898)
  line L588 (0.0465, 0.2898) -> (0.0406, 0.2906)
  line L589 (0.0406, 0.2906) -> (0.0347, 0.2915)
  line L590 (0.0347, 0.2915) -> (0.0287, 0.2927)
  line L591 (0.0287, 0.2927) -> (0.0227, 0.2941)
  line L592 (0.0227, 0.2941) -> (0.0167, 0.2957)
  line L593 (0.0167, 0.2957) -> (0.0055, 0.3447)
  line L594 (0.0055, 0.3447) -> (0.0102, 0.3488)
  line L595 (0.0102, 0.3488) -> (0.015, 0.3527)
  line L596 (0.015, 0.3527) -> (0.0199, 0.3563)
  line L597 (0.0199, 0.3563) -> (0.0248, 0.3598)
  line L598 (0.0248, 0.3598) -> (0.0298, 0.363)
  line L599 (0.0298, 0.363) -> (0.0348, 0.366)
  line L600 (0.0348, 0.366) -> (0.0398, 0.3688)
  line L601 (0.0398, 0.3688) -> (0.0449, 0.3714)
  line L602 (0.0449, 0.3714) -> (0.05, 0.3736)
  line L603 (0.05, 0.3736) -> (0.0552, 0.3755)
  line L604 (0.0552, 0.3755) -> (0.0604, 0.3771)
  line L605 (0.0604, 0.3771) -> (0.0656, 0.3782)
  line L606 (0.0656, 0.3782) -> (0.0682, 0.3788)
  line L607 (0.0682, 0.3788) -> (0.0708, 0.3796)
  line L608 (0.0708, 0.3796) -> (0.0734, 0.3807)
  line L609 (0.0734, 0.3807) -> (0.0747, 0.3813)
  line L610 (0.0747, 0.3813) -> (0.076, 0.3821)
  line L611 (0.076, 0.3821) -> (0.0772, 0.383)
  line L612 (0.0772, 0.383) -> (0.0785, 0.3841)
  line L613 (0.0785, 0.3841) -> (0.0797, 0.3855)
  line L614 (0.0797, 0.3855) -> (0.0808, 0.3892)
  line L615 (0.0808, 0.3892) -> (0.0808, 0.4341)
  line L616 (0.4842, 0.4117) -> (0.4817, 0.4304)
  line L617 (0.4817, 0.4304) -> (0.4745, 0.4479)
  line L618 (0.4745, 0.4479) -> (0.4629, 0.4629)
  line L619 (0.4629, 0.4629) -> (0.4479, 0.4745)
  line L620 (0.4479, 0.4745) -> (0.4304, 0.4817)
  line L621 (0.4304, 0.4817) -> (0.4117, 0.4842)
  line L622 (0.4117, 0.4842) -> (0.3929, 0.4817)
  line L623 (0.3929, 0.4817) -> (0.3754, 0.4745)
  line L624 (0.3754, 0.4745) -> (0.3604, 0.4629)
  line L625 (0.3604, 0.4629) -> (0.3489, 0.4479)
  line L626 (0.3489, 0.4479) -> (0.3416, 0.4304)
  line L627 (0.3416, 0.4304) -> (0.3392, 0.4117)
  line L628 (0.3392, 0.4117) -> (0.3416, 0.3929)
  line L629 (0.3416, 0.3929) -> (0.3489, 0.3754)
  line L630 (0.3489, 0.3754) -> (0.3604, 0.3604)
  line L631 (0.3604, 0.3604) -> (0.3754, 0.3489)
  line L632 (0.3754, 0.3489) -> (0.3929, 0.3416)
  line L633 (0.3929, 0.3416) -> (0.4117, 0.3392)
  line L634 (0.4117, 0.3392) -> (0.4304, 0.3416)
  line L635 (0.4304, 0.3416) -> (0.4479, 0.3489)
  line L636 (0.4479, 0.3489) -> (0.4629, 0.3604)
  line L637 (0.4629, 0.3604) -> (0.4745, 0.3754)
  line L638 (0.4745, 0.3754) -> (0.4817, 0.3929)
  line L639 (0.4817, 0.3929) -> (0.4842, 0.4117)
  point P0 (0, 0)
  constraints: 1280 end point
extrude "Extrusion1" add sketch "Sketch1" along normal blind 1
sketch "Sketch2" plane through (0, 1, 0) normal (0, 1, 0) x (1, 0, 0)
  line L0 (-0.4842, -0.4117) -> (-0.4817, -0.3929)
  line L1 (-0.4817, -0.3929) -> (-0.4745, -0.3754)
  line L2 (-0.4745, -0.3754) -> (-0.4629, -0.3604)
  line L3 (-0.4629, -0.3604) -> (-0.4479, -0.3489)
  line L4 (-0.4479, -0.3489) -> (-0.4304, -0.3416)
  line L5 (-0.4304, -0.3416) -> (-0.4117, -0.3392)
  line L6 (-0.4117, -0.3392) -> (-0.3929, -0.3416)
  line L7 (-0.3929, -0.3416) -> (-0.3754, -0.3489)
  line L8 (-0.3754, -0.3489) -> (-0.3604, -0.3604)
  line L9 (-0.3604, -0.3604) -> (-0.3489, -0.3754)
  line L10 (-0.3489, -0.3754) -> (-0.3416, -0.3929)
  line L11 (-0.3416, -0.3929) -> (-0.3392, -0.4117)
  line L12 (-0.3392, -0.4117) -> (-0.3416, -0.4304)
  line L13 (-0.3416, -0.4304) -> (-0.3489, -0.4479)
  line L14 (-0.3489, -0.4479) -> (-0.3604, -0.4629)
  line L15 (-0.3604, -0.4629) -> (-0.3754, -0.4745)
  line L16 (-0.3754, -0.4745) -> (-0.3929, -0.4817)
  line L17 (-0.3929, -0.4817) -> (-0.4117, -0.4842)
  line L18 (-0.4117, -0.4842) -> (-0.4304, -0.4817)
  line L19 (-0.4304, -0.4817) -> (-0.4479, -0.4745)
  line L20 (-0.4479, -0.4745) -> (-0.4629, -0.4629)
  line L21 (-0.4629, -0.4629) -> (-0.4745, -0.4479)
  line L22 (-0.4745, -0.4479) -> (-0.4817, -0.4304)
  line L23 (-0.4817, -0.4304) -> (-0.4842, -0.4117)
  line L24 (-0.0797, -0.4378) -> (-0.0808, -0.4341)
  line L25 (-0.0808, -0.4341) -> (-0.0808, -0.3892)
  line L26 (-0.0808, -0.3892) -> (-0.0797, -0.3855)
  line L27 (-0.0797, -0.3855) -> (-0.0785, -0.3841)
  line L28 (-0.0785, -0.3841) -> (-0.0772, -0.383)
  line L29 (-0.0772, -0.383) -> (-0.076, -0.3821)
  line L30 (-0.076, -0.3821) -> (-0.0747, -0.3813)
  line L31 (-0.0747, -0.3813) -> (-0.0734, -0.3807)
  line L32 (-0.0734, -0.3807) -> (-0.0708, -0.3796)
  line L33 (-0.0708, -0.3796) -> (-0.0682, -0.3788)
  line L34 (-0.0682, -0.3788) -> (-0.0656, -0.3782)
  line L35 (-0.0656, -0.3782) -> (-0.0604, -0.3771)
  line L36 (-0.0604, -0.3771) -> (-0.0552, -0.3755)
  line L37 (-0.0552, -0.3755) -> (-0.05, -0.3736)
  line L38 (-0.05, -0.3736) -> (-0.0449, -0.3714)
  line L39 (-0.0449, -0.3714) -> (-0.0398, -0.3688)
  line L40 (-0.0398, -0.3688) -> (-0.0348, -0.366)
  line L41 (-0.0348, -0.366) -> (-0.0298, -0.363)
  line L42 (-0.0298, -0.363) -> (-0.0248, -0.3598)
  line L43 (-0.0248, -0.3598) -> (-0.0199, -0.3563)
  line L44 (-0.0199, -0.3563) -> (-0.015, -0.3527)
  line L45 (-0.015, -0.3527) -> (-0.0102, -0.3488)
  line L46 (-0.0102, -0.3488) -> (-0.0055, -0.3447)
  line L47 (-0.0055, -0.3447) -> (-0.0167, -0.2957)
  line L48 (-0.0167, -0.2957) -> (-0.0227, -0.2941)
  line L49 (-0.0227, -0.2941) -> (-0.0287, -0.2927)
  line L50 (-0.0287, -0.2927) -> (-0.0347, -0.2915)
  line L51 (-0.0347, -0.2915) -> (-0.0406, -0.2906)
  line L52 (-0.0406, -0.2906) -> (-0.0465, -0.2898)
  line L53 (-0.0465, -0.2898) -> (-0.0523, -0.2892)
  line L54 (-0.0523, -0.2892) -> (-0.058, -0.2889)
  line L55 (-0.058, -0.2889) -> (-0.0637, -0.2888)
  line L56 (-0.0637, -0.2888) -> (-0.0693, -0.289)
  line L57 (-0.0693, -0.289) -> (-0.0748, -0.2895)
  line L58 (-0.0748, -0.2895) -> (-0.0802, -0.2904)
  line L59 (-0.0802, -0.2904) -> (-0.0854, -0.2917)
  line L60 (-0.0854, -0.2917) -> (-0.088, -0.2923)
  line L61 (-0.088, -0.2923) -> (-0.0907, -0.2927)
  line L62 (-0.0907, -0.2927) -> (-0.0935, -0.2928)
  line L63 (-0.0935, -0.2928) -> (-0.0949, -0.2928)
  line L64 (-0.0949, -0.2928) -> (-0.0964, -0.2927)
  line L65 (-0.0964, -0.2927) -> (-0.0979, -0.2924)
  line L66 (-0.0979, -0.2924) -> (-0.0995, -0.292)
  line L67 (-0.0995, -0.292) -> (-0.1012, -0.2912)
  line L68 (-0.1012, -0.2912) -> (-0.1038, -0.2883)
  line L69 (-0.1038, -0.2883) -> (-0.1233, -0.2479)
  line L70 (-0.1233, -0.2479) -> (-0.1239, -0.2441)
  line L71 (-0.1239, -0.2441) -> (-0.1235, -0.2422)
  line L72 (-0.1235, -0.2422) -> (-0.1228, -0.2407)
  line L73 (-0.1228, -0.2407) -> (-0.1221, -0.2394)
  line L74 (-0.1221, -0.2394) -> (-0.1212, -0.2381)
  line L75 (-0.1212, -0.2381) -> (-0.1204, -0.237)
  line L76 (-0.1204, -0.237) -> (-0.1185, -0.2349)
  line L77 (-0.1185, -0.2349) -> (-0.1165, -0.2331)
  line L78 (-0.1165, -0.2331) -> (-0.1144, -0.2314)
  line L79 (-0.1144, -0.2314) -> (-0.1102, -0.2281)
  line L80 (-0.1102, -0.2281) -> (-0.1061, -0.2244)
  line L81 (-0.1061, -0.2244) -> (-0.1023, -0.2205)
  line L82 (-0.1023, -0.2205) -> (-0.0987, -0.2162)
  line L83 (-0.0987, -0.2162) -> (-0.0952, -0.2117)
  line L84 (-0.0952, -0.2117) -> (-0.0919, -0.207)
  line L85 (-0.0919, -0.207) -> (-0.0887, -0.2021)
  line L86 (-0.0887, -0.2021) -> (-0.0856, -0.1971)
  line L87 (-0.0856, -0.1971) -> (-0.0827, -0.1918)
  line L88 (-0.0827, -0.1918) -> (-0.0799, -0.1864)
  line L89 (-0.0799, -0.1864) -> (-0.0773, -0.1809)
  line L90 (-0.0773, -0.1809) -> (-0.0747, -0.1751)
  line L91 (-0.0747, -0.1751) -> (-0.1061, -0.1358)
  line L92 (-0.1061, -0.1358) -> (-0.1122, -0.137)
  line L93 (-0.1122, -0.137) -> (-0.1182, -0.1384)
  line L94 (-0.1182, -0.1384) -> (-0.1241, -0.1399)
  line L95 (-0.1241, -0.1399) -> (-0.1299, -0.1416)
  line L96 (-0.1299, -0.1416) -> (-0.1355, -0.1434)
  line L97 (-0.1355, -0.1434) -> (-0.141, -0.1454)
  line L98 (-0.141, -0.1454) -> (-0.1463, -0.1476)
  line L99 (-0.1463, -0.1476) -> (-0.1515, -0.15)
  line L100 (-0.1515, -0.15) -> (-0.1564, -0.1526)
  line L101 (-0.1564, -0.1526) -> (-0.1612, -0.1555)
  line L102 (-0.1612, -0.1555) -> (-0.1656, -0.1586)
  line L103 (-0.1656, -0.1586) -> (-0.1697, -0.162)
  line L104 (-0.1697, -0.162) -> (-0.1719, -0.1637)
  line L105 (-0.1719, -0.1637) -> (-0.1741, -0.1652)
  line L106 (-0.1741, -0.1652) -> (-0.1766, -0.1665)
  line L107 (-0.1766, -0.1665) -> (-0.1779, -0.1671)
  line L108 (-0.1779, -0.1671) -> (-0.1792, -0.1677)
  line L109 (-0.1792, -0.1677) -> (-0.1807, -0.1681)
  line L110 (-0.1807, -0.1681) -> (-0.1823, -0.1684)
  line L111 (-0.1823, -0.1684) -> (-0.1843, -0.1684)
  line L112 (-0.1843, -0.1684) -> (-0.1878, -0.167)
  line L113 (-0.1878, -0.167) -> (-0.2229, -0.1389)
  line L114 (-0.2229, -0.1389) -> (-0.2251, -0.1358)
  line L115 (-0.2251, -0.1358) -> (-0.2255, -0.134)
  line L116 (-0.2255, -0.134) -> (-0.2256, -0.1323)
  line L117 (-0.2256, -0.1323) -> (-0.2255, -0.1308)
  line L118 (-0.2255, -0.1308) -> (-0.2253, -0.1293)
  line L119 (-0.2253, -0.1293) -> (-0.225, -0.1279)
  line L120 (-0.225, -0.1279) -> (-0.2242, -0.1252)
  line L121 (-0.2242, -0.1252) -> (-0.2232, -0.1227)
  line L122 (-0.2232, -0.1227) -> (-0.2221, -0.1203)
  line L123 (-0.2221, -0.1203) -> (-0.2197, -0.1155)
  line L124 (-0.2197, -0.1155) -> (-0.2176, -0.1104)
  line L125 (-0.2176, -0.1104) -> (-0.2159, -0.1052)
  line L126 (-0.2159, -0.1052) -> (-0.2145, -0.0998)
  line L127 (-0.2145, -0.0998) -> (-0.2133, -0.0942)
  line L128 (-0.2133, -0.0942) -> (-0.2123, -0.0885)
  line L129 (-0.2123, -0.0885) -> (-0.2116, -0.0828)
  line L130 (-0.2116, -0.0828) -> (-0.211, -0.0768)
  line L131 (-0.211, -0.0768) -> (-0.2107, -0.0709)
  line L132 (-0.2107, -0.0709) -> (-0.2105, -0.0648)
  line L133 (-0.2105, -0.0648) -> (-0.2105, -0.0586)
  line L134 (-0.2105, -0.0586) -> (-0.2107, -0.0524)
  line L135 (-0.2107, -0.0524) -> (-0.256, -0.0306)
  line L136 (-0.256, -0.0306) -> (-0.261, -0.0343)
  line L137 (-0.261, -0.0343) -> (-0.2659, -0.0381)
  line L138 (-0.2659, -0.0381) -> (-0.2705, -0.042)
  line L139 (-0.2705, -0.042) -> (-0.275, -0.046)
  line L140 (-0.275, -0.046) -> (-0.2793, -0.0501)
  line L141 (-0.2793, -0.0501) -> (-0.2833, -0.0544)
  line L142 (-0.2833, -0.0544) -> (-0.2872, -0.0587)
  line L143 (-0.2872, -0.0587) -> (-0.2908, -0.063)
  line L144 (-0.2908, -0.063) -> (-0.2941, -0.0675)
  line L145 (-0.2941, -0.0675) -> (-0.2971, -0.0721)
  line L146 (-0.2971, -0.0721) -> (-0.2998, -0.0769)
  line L147 (-0.2998, -0.0769) -> (-0.302, -0.0818)
  line L148 (-0.302, -0.0818) -> (-0.3032, -0.0842)
  line L149 (-0.3032, -0.0842) -> (-0.3046, -0.0865)
  line L150 (-0.3046, -0.0865) -> (-0.3062, -0.0888)
  line L151 (-0.3062, -0.0888) -> (-0.3071, -0.0899)
  line L152 (-0.3071, -0.0899) -> (-0.3081, -0.091)
  line L153 (-0.3081, -0.091) -> (-0.3093, -0.092)
  line L154 (-0.3093, -0.092) -> (-0.3106, -0.093)
  line L155 (-0.3106, -0.093) -> (-0.3123, -0.0938)
  line L156 (-0.3123, -0.0938) -> (-0.3161, -0.0941)
  line L157 (-0.3161, -0.0941) -> (-0.3599, -0.0841)
  line L158 (-0.3599, -0.0841) -> (-0.3633, -0.0822)
  line L159 (-0.3633, -0.0822) -> (-0.3644, -0.0807)
  line L160 (-0.3644, -0.0807) -> (-0.3652, -0.0792)
  line L161 (-0.3652, -0.0792) -> (-0.3658, -0.0778)
  line L162 (-0.3658, -0.0778) -> (-0.3663, -0.0764)
  line L163 (-0.3663, -0.0764) -> (-0.3666, -0.075)
  line L164 (-0.3666, -0.075) -> (-0.367, -0.0723)
  line L165 (-0.367, -0.0723) -> (-0.3673, -0.0695)
  line L166 (-0.3673, -0.0695) -> (-0.3673, -0.0669)
  line L167 (-0.3673, -0.0669) -> (-0.3672, -0.0615)
  line L168 (-0.3672, -0.0615) -> (-0.3676, -0.0561)
  line L169 (-0.3676, -0.0561) -> (-0.3683, -0.0506)
  line L170 (-0.3683, -0.0506) -> (-0.3694, -0.0451)
  line L171 (-0.3694, -0.0451) -> (-0.3707, -0.0396)
  line L172 (-0.3707, -0.0396) -> (-0.3723, -0.034)
  line L173 (-0.3723, -0.034) -> (-0.3741, -0.0285)
  line L174 (-0.3741, -0.0285) -> (-0.3762, -0.0229)
  line L175 (-0.3762, -0.0229) -> (-0.3784, -0.0174)
  line L176 (-0.3784, -0.0174) -> (-0.3809, -0.0118)
  line L177 (-0.3809, -0.0118) -> (-0.3836, -0.0063)
  line L178 (-0.3836, -0.0063) -> (-0.3865, -0.0008)
  line L179 (-0.3865, -0.0008) -> (-0.4368, -0.0008)
  line L180 (-0.4368, -0.0008) -> (-0.4397, -0.0063)
  line L181 (-0.4397, -0.0063) -> (-0.4424, -0.0118)
  line L182 (-0.4424, -0.0118) -> (-0.4449, -0.0174)
  line L183 (-0.4449, -0.0174) -> (-0.4472, -0.0229)
  line L184 (-0.4472, -0.0229) -> (-0.4492, -0.0285)
  line L185 (-0.4492, -0.0285) -> (-0.4511, -0.034)
  line L186 (-0.4511, -0.034) -> (-0.4526, -0.0396)
  line L187 (-0.4526, -0.0396) -> (-0.454, -0.0451)
  line L188 (-0.454, -0.0451) -> (-0.455, -0.0506)
  line L189 (-0.455, -0.0506) -> (-0.4558, -0.0561)
  line L190 (-0.4558, -0.0561) -> (-0.4561, -0.0615)
  line L191 (-0.4561, -0.0615) -> (-0.456, -0.0669)
  line L192 (-0.456, -0.0669) -> (-0.4561, -0.0695)
  line L193 (-0.4561, -0.0695) -> (-0.4563, -0.0723)
  line L194 (-0.4563, -0.0723) -> (-0.4567, -0.075)
  line L195 (-0.4567, -0.075) -> (-0.4571, -0.0764)
  line L196 (-0.4571, -0.0764) -> (-0.4575, -0.0778)
  line L197 (-0.4575, -0.0778) -> (-0.4581, -0.0792)
  line L198 (-0.4581, -0.0792) -> (-0.4589, -0.0807)
  line L199 (-0.4589, -0.0807) -> (-0.4601, -0.0822)
  line L200 (-0.4601, -0.0822) -> (-0.4634, -0.0841)
  line L201 (-0.4634, -0.0841) -> (-0.5072, -0.0941)
  line L202 (-0.5072, -0.0941) -> (-0.511, -0.0938)
  line L203 (-0.511, -0.0938) -> (-0.5127, -0.093)
  line L204 (-0.5127, -0.093) -> (-0.5141, -0.092)
  line L205 (-0.5141, -0.092) -> (-0.5152, -0.091)
  line L206 (-0.5152, -0.091) -> (-0.5162, -0.0899)
  line L207 (-0.5162, -0.0899) -> (-0.5171, -0.0888)
  line L208 (-0.5171, -0.0888) -> (-0.5187, -0.0865)
  line L209 (-0.5187, -0.0865) -> (-0.5201, -0.0842)
  line L210 (-0.5201, -0.0842) -> (-0.5213, -0.0818)
  line L211 (-0.5213, -0.0818) -> (-0.5235, -0.0769)
  line L212 (-0.5235, -0.0769) -> (-0.5262, -0.0721)
  line L213 (-0.5262, -0.0721) -> (-0.5292, -0.0675)
  line L214 (-0.5292, -0.0675) -> (-0.5326, -0.063)
  line L215 (-0.5326, -0.063) -> (-0.5362, -0.0587)
  line L216 (-0.5362, -0.0587) -> (-0.54, -0.0544)
  line L217 (-0.54, -0.0544) -> (-0.5441, -0.0501)
  line L218 (-0.5441, -0.0501) -> (-0.5483, -0.046)
  line L219 (-0.5483, -0.046) -> (-0.5528, -0.042)
  line L220 (-0.5528, -0.042) -> (-0.5575, -0.0381)
  line L221 (-0.5575, -0.0381) -> (-0.5623, -0.0343)
  line L222 (-0.5623, -0.0343) -> (-0.5673, -0.0306)
  line L223 (-0.5673, -0.0306) -> (-0.6126, -0.0524)
  line L224 (-0.6126, -0.0524) -> (-0.6128, -0.0586)
  line L225 (-0.6128, -0.0586) -> (-0.6128, -0.0648)
  line L226 (-0.6128, -0.0648) -> (-0.6127, -0.0709)
  line L227 (-0.6127, -0.0709) -> (-0.6123, -0.0768)
  line L228 (-0.6123, -0.0768) -> (-0.6118, -0.0828)
  line L229 (-0.6118, -0.0828) -> (-0.611, -0.0885)
  line L230 (-0.611, -0.0885) -> (-0.61, -0.0942)
  line L231 (-0.61, -0.0942) -> (-0.6088, -0.0998)
  line L232 (-0.6088, -0.0998) -> (-0.6074, -0.1052)
  line L233 (-0.6074, -0.1052) -> (-0.6057, -0.1104)
  line L234 (-0.6057, -0.1104) -> (-0.6037, -0.1155)
  line L235 (-0.6037, -0.1155) -> (-0.6012, -0.1203)
  line L236 (-0.6012, -0.1203) -> (-0.6001, -0.1227)
  line L237 (-0.6001, -0.1227) -> (-0.5991, -0.1252)
  line L238 (-0.5991, -0.1252) -> (-0.5983, -0.1279)
  line L239 (-0.5983, -0.1279) -> (-0.598, -0.1293)
  line L240 (-0.598, -0.1293) -> (-0.5978, -0.1308)
  line L241 (-0.5978, -0.1308) -> (-0.5977, -0.1323)
  line L242 (-0.5977, -0.1323) -> (-0.5978, -0.134)
  line L243 (-0.5978, -0.134) -> (-0.5982, -0.1358)
  line L244 (-0.5982, -0.1358) -> (-0.6004, -0.1389)
  line L245 (-0.6004, -0.1389) -> (-0.6355, -0.167)
  line L246 (-0.6355, -0.167) -> (-0.6391, -0.1684)
  line L247 (-0.6391, -0.1684) -> (-0.641, -0.1684)
  line L248 (-0.641, -0.1684) -> (-0.6426, -0.1681)
  line L249 (-0.6426, -0.1681) -> (-0.6441, -0.1677)
  line L250 (-0.6441, -0.1677) -> (-0.6455, -0.1671)
  line L251 (-0.6455, -0.1671) -> (-0.6468, -0.1665)
  line L252 (-0.6468, -0.1665) -> (-0.6492, -0.1652)
  line L253 (-0.6492, -0.1652) -> (-0.6515, -0.1637)
  line L254 (-0.6515, -0.1637) -> (-0.6536, -0.162)
  line L255 (-0.6536, -0.162) -> (-0.6577, -0.1586)
  line L256 (-0.6577, -0.1586) -> (-0.6622, -0.1555)
  line L257 (-0.6622, -0.1555) -> (-0.6669, -0.1526)
  line L258 (-0.6669, -0.1526) -> (-0.6719, -0.15)
  line L259 (-0.6719, -0.15) -> (-0.677, -0.1476)
  line L260 (-0.677, -0.1476) -> (-0.6823, -0.1454)
  line L261 (-0.6823, -0.1454) -> (-0.6878, -0.1434)
  line L262 (-0.6878, -0.1434) -> (-0.6934, -0.1416)
  line L263 (-0.6934, -0.1416) -> (-0.6992, -0.1399)
  line L264 (-0.6992, -0.1399) -> (-0.7051, -0.1384)
  line L265 (-0.7051, -0.1384) -> (-0.7111, -0.137)
  line L266 (-0.7111, -0.137) -> (-0.7172, -0.1358)
  line L267 (-0.7172, -0.1358) -> (-0.7486, -0.1751)
  line L268 (-0.7486, -0.1751) -> (-0.7461, -0.1809)
  line L269 (-0.7461, -0.1809) -> (-0.7434, -0.1864)
  line L270 (-0.7434, -0.1864) -> (-0.7406, -0.1918)
  line L271 (-0.7406, -0.1918) -> (-0.7377, -0.1971)
  line L272 (-0.7377, -0.1971) -> (-0.7347, -0.2021)
  line L273 (-0.7347, -0.2021) -> (-0.7315, -0.207)
  line L274 (-0.7315, -0.207) -> (-0.7281, -0.2117)
  line L275 (-0.7281, -0.2117) -> (-0.7246, -0.2162)
  line L276 (-0.7246, -0.2162) -> (-0.721, -0.2205)
  line L277 (-0.721, -0.2205) -> (-0.7172, -0.2244)
  line L278 (-0.7172, -0.2244) -> (-0.7132, -0.2281)
  line L279 (-0.7132, -0.2281) -> (-0.7089, -0.2314)
  line L280 (-0.7089, -0.2314) -> (-0.7068, -0.2331)
  line L281 (-0.7068, -0.2331) -> (-0.7048, -0.2349)
  line L282 (-0.7048, -0.2349) -> (-0.703, -0.237)
  line L283 (-0.703, -0.237) -> (-0.7021, -0.2381)
  line L284 (-0.7021, -0.2381) -> (-0.7013, -0.2394)
  line L285 (-0.7013, -0.2394) -> (-0.7005, -0.2407)
  line L286 (-0.7005, -0.2407) -> (-0.6999, -0.2422)
  line L287 (-0.6999, -0.2422) -> (-0.6994, -0.2441)
  line L288 (-0.6994, -0.2441) -> (-0.7, -0.2479)
  line L289 (-0.7, -0.2479) -> (-0.7195, -0.2883)
  line L290 (-0.7195, -0.2883) -> (-0.7221, -0.2912)
  line L291 (-0.7221, -0.2912) -> (-0.7238, -0.292)
  line L292 (-0.7238, -0.292) -> (-0.7254, -0.2924)
  line L293 (-0.7254, -0.2924) -> (-0.7269, -0.2927)
  line L294 (-0.7269, -0.2927) -> (-0.7284, -0.2928)
  line L295 (-0.7284, -0.2928) -> (-0.7299, -0.2928)
  line L296 (-0.7299, -0.2928) -> (-0.7326, -0.2927)
  line L297 (-0.7326, -0.2927) -> (-0.7353, -0.2923)
  line L298 (-0.7353, -0.2923) -> (-0.738, -0.2917)
  line L299 (-0.738, -0.2917) -> (-0.7432, -0.2904)
  line L300 (-0.7432, -0.2904) -> (-0.7485, -0.2895)
  line L301 (-0.7485, -0.2895) -> (-0.754, -0.289)
  line L302 (-0.754, -0.289) -> (-0.7596, -0.2888)
  line L303 (-0.7596, -0.2888) -> (-0.7653, -0.2889)
  line L304 (-0.7653, -0.2889) -> (-0.771, -0.2892)
  line L305 (-0.771, -0.2892) -> (-0.7769, -0.2898)
  line L306 (-0.7769, -0.2898) -> (-0.7827, -0.2906)
  line L307 (-0.7827, -0.2906) -> (-0.7887, -0.2915)
  line L308 (-0.7887, -0.2915) -> (-0.7946, -0.2927)
  line L309 (-0.7946, -0.2927) -> (-0.8006, -0.2941)
  line L310 (-0.8006, -0.2941) -> (-0.8067, -0.2957)
  line L311 (-0.8067, -0.2957) -> (-0.8178, -0.3447)
  line L312 (-0.8178, -0.3447) -> (-0.8131, -0.3488)
  line L313 (-0.8131, -0.3488) -> (-0.8083, -0.3527)
  line L314 (-0.8083, -0.3527) -> (-0.8034, -0.3563)
  line L315 (-0.8034, -0.3563) -> (-0.7985, -0.3598)
  line L316 (-0.7985, -0.3598) -> (-0.7936, -0.363)
  line L317 (-0.7936, -0.363) -> (-0.7886, -0.366)
  line L318 (-0.7886, -0.366) -> (-0.7835, -0.3688)
  line L319 (-0.7835, -0.3688) -> (-0.7784, -0.3714)
  line L320 (-0.7784, -0.3714) -> (-0.7733, -0.3736)
  line L321 (-0.7733, -0.3736) -> (-0.7682, -0.3755)
  line L322 (-0.7682, -0.3755) -> (-0.763, -0.3771)
  line L323 (-0.763, -0.3771) -> (-0.7577, -0.3782)
  line L324 (-0.7577, -0.3782) -> (-0.7551, -0.3788)
  line L325 (-0.7551, -0.3788) -> (-0.7525, -0.3796)
  line L326 (-0.7525, -0.3796) -> (-0.7499, -0.3807)
  line L327 (-0.7499, -0.3807) -> (-0.7486, -0.3813)
  line L328 (-0.7486, -0.3813) -> (-0.7473, -0.3821)
  line L329 (-0.7473, -0.3821) -> (-0.7461, -0.383)
  line L330 (-0.7461, -0.383) -> (-0.7449, -0.3841)
  line L331 (-0.7449, -0.3841) -> (-0.7436, -0.3855)
  line L332 (-0.7436, -0.3855) -> (-0.7426, -0.3892)
  line L333 (-0.7426, -0.3892) -> (-0.7426, -0.4341)
  line L334 (-0.7426, -0.4341) -> (-0.7436, -0.4378)
  line L335 (-0.7436, -0.4378) -> (-0.7449, -0.4393)
  line L336 (-0.7449, -0.4393) -> (-0.7461, -0.4404)
  line L337 (-0.7461, -0.4404) -> (-0.7473, -0.4413)
  line L338 (-0.7473, -0.4413) -> (-0.7486, -0.442)
  line L339 (-0.7486, -0.442) -> (-0.7499, -0.4426)
  line L340 (-0.7499, -0.4426) -> (-0.7525, -0.4437)
  line L341 (-0.7525, -0.4437) -> (-0.7551, -0.4445)
  line L342 (-0.7551, -0.4445) -> (-0.7577, -0.4451)
  line L343 (-0.7577, -0.4451) -> (-0.763, -0.4462)
  line L344 (-0.763, -0.4462) -> (-0.7682, -0.4478)
  line L345 (-0.7682, -0.4478) -> (-0.7733, -0.4497)
  line L346 (-0.7733, -0.4497) -> (-0.7784, -0.452)
  line L347 (-0.7784, -0.452) -> (-0.7835, -0.4545)